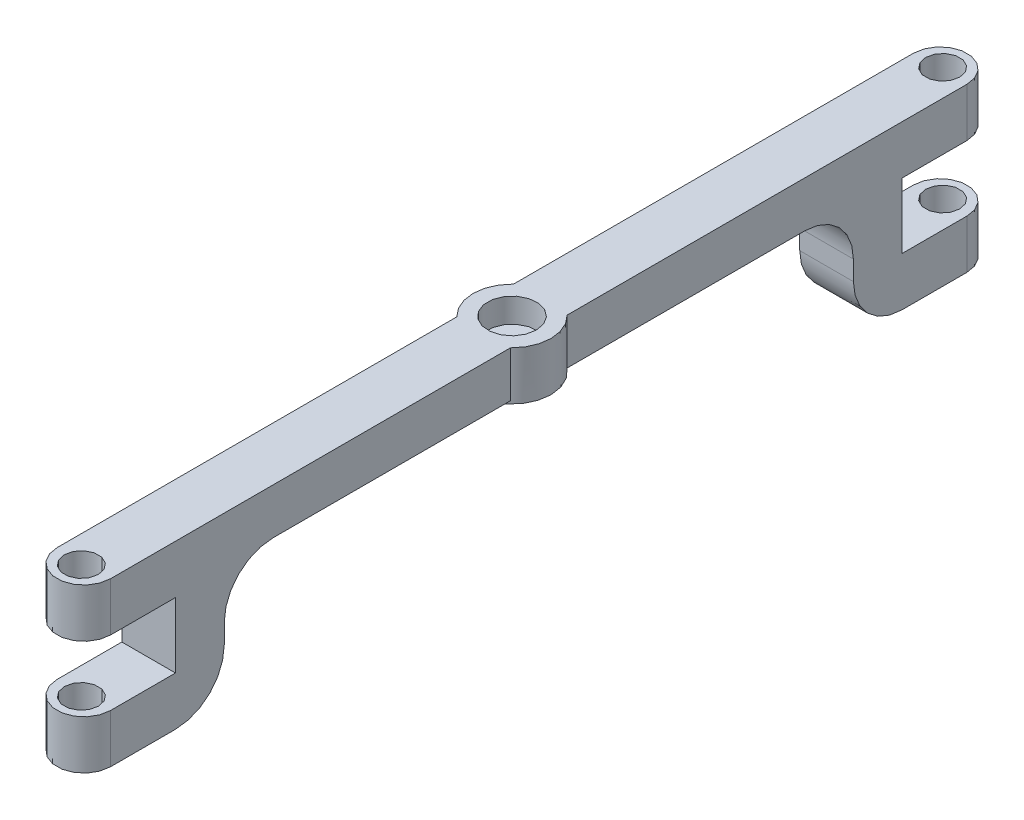
# Autodesk Inventor part: Балка рулевого управления
Saved by Autodesk Inventor 2020 (Build 240168000, 168)
## iProperties
Created: 2021-03-21
Part Number: Балка рулевого управления
Material: Типовые
Document SubType Name: Modeling
Designer: Антон
Density: 1 g/cm^3
Appearance: По умолчанию
Author: Антон
Autodesk Inventor part; units mm, degrees
ref_plane "YZ Plane" through (0, 0, 0) normal (1, 0, 0) x (0, 1, 0)
ref_plane "XZ Plane" through (0, 0, 0) normal (0, 1, 0) x (-1, 0, 0)
ref_plane "XY Plane" through (0, 0, 0) normal (0, 0, 1) x (1, 0, 0)
sketch "Эскиз1" plane through (0, 0, 0) normal (0, 1, 0) x (-1, 0, 0)
  line L0 (0, 0) -> (5.5, 0)
  line L1 (5.5, 0) -> (5.5, -46.65)
  line L2 (5.5, -46.65) -> (0, -46.65)
  line L3 (0, -46.65) -> (0, 0)
  line L4 (2.75, 0) -> (2.75, -2.5)
  circle A0 centre (2.75, -2.5) radius 1.75
  dimension "d0" = 5.5
  dimension "d1" = 46.65
  dimension "d4" = 2.5
  dimension "d5" = 3.5
  constraints: 10 end point, 2 parallel, 1 centre point, 1 coincident, 1 horizontal, 1 midpoint, 1 perpendicular, 1 vertical
  measures "d0" distance of L1.end L2.end
  measures "d1" distance of L0.end L1.end
  measures "d4" distance of L4.start L4.end
  measures "d5" diameter of A0
extrude "Выдавливание1" add sketch "Эскиз1" along normal blind 5
fillet "Сопряжение1" radius 2.75 2 edges at (0, 2.5, 0) (-5.5, 2.5, 0)
sketch "Эскиз2" plane through (0, 5, 0) normal (0, 1, 0) x (1, 0, 0)
  line L0 (0, 2.75) -> (0, 46.65) projected
  line L1 (-5.5, 46.65) -> (0, 46.65)
  line L2 (0, 46.65) -> (0, 9.4)
  line L3 (0, 9.4) -> (-5.5, 9.4)
  line L4 (-5.5, 9.4) -> (-5.5, 46.65)
  point P0 (0, 0)
  point P1 (0, 46.65)
  dimension "d7" = 37.25
  dimension "d45" = 43.9
  constraints: 8 end point, 2 parallel, 1 horizontal, 1 perpendicular, 1 point on line
  measures "d7" distance of L1.end L2.end
  measures "d45" distance of L0.start L0.end
extrude "Выдавливание2" add sketch "Эскиз2" along normal blind 3.35
mirror "Зеркальное отражение3" about plane through (-2.75, 8.35, -28.025) normal (0, 1, 0)
sketch "Эскиз8" plane through (0, 0, -2.75) normal (1, 0, 0) x (0, 0, -1)
  line L0 (0, 0) -> (43.9, 0) projected
  line L1 (43.9, 0) -> (11.65, 0)
  line L2 (11.65, 0) -> (11.65, 12)
  line L3 (11.65, 12) -> (43.9, 12)
  line L4 (43.9, 12) -> (43.9, 0)
  line L5 (6.65, 5) -> (6.65, 11.7) projected
  point P0 (-2.75, 0)
  dimension "d35" = 32.25
  dimension "d36" = 12
  dimension "d52" = 37.25
  constraints: 6 end point, 2 horizontal, 1 parallel, 1 perpendicular, 3 other
  measures "d35" distance of L2.end L4.start
  measures "d36" distance of L1.end L2.end
  measures "d52" distance between parallel lines of L4 L5
extrude "Выдавливание6" cut sketch "Эскиз8" against normal through all
mirror "Зеркальное отражение6" about plane through (0, 0, -46.65) normal (0, 0, -1)
fillet "Сопряжение5" radius 5 4 edges at (-2.75, 12, -14.4) (-2.75, 0, -14.4) (-2.75, 0, -78.9) (-2.75, 12, -78.9)
sketch "Эскиз9" plane through (-2.75, 16.7, -2.75) normal (0, 1, 0) x (1, 0, 0)
  line L0 (2.75, 87.8) -> (2.75, 0) projected
  line L1 (2.75, 43.9) -> (-2.75, 43.9)
  line L2 (-2.75, 87.8) -> (-2.75, 0) projected
  circle A0 centre (0, 43.9) radius 4
  point P0 (2.75, -2.75)
  point P1 (-2.75, 87.8)
  point P2 (-2.75, 0)
  point P3 (60.3162, 64.5588)
  point P4 (-2.1213, 2.1213)
  dimension "d46" = 8
  constraints: 2 end point, 2 midpoint, 1 centre point, 2 other
  measures "d46" diameter of A0
extrude "Выдавливание7" add sketch "Эскиз9" against normal blind 5
sketch "Эскиз10" plane through (-2.75, 16.7, -2.75) normal (0, 1, 0) x (1, 0, 0)
  arc A0 (-2.75, 46.8047) -> (-2.75, 40.9953) centre (0, 43.9) ccw projected
  arc A1 (2.75, 40.9953) -> (2.75, 46.8047) centre (0, 43.9) ccw projected
  circle A2 centre (0, 43.9) radius 2.5
  point P0 (2.75, -2.75)
  dimension "d49" = 5
  constraints: 1 centre point, 1 coincident
  measures "d49" diameter of A2
extrude "Выдавливание8" cut sketch "Эскиз10" against normal blind 2.5
